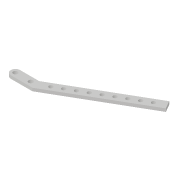
# Autodesk Inventor part: CollectorArmParametric
Saved by Autodesk Inventor 2018 (Build 220112000, 112)
## iProperties
Created: 2018-12-15
Part Number: CollectorArmParametric
Material: Generic
Document SubType Name: Modeling
Designer: ball
Density: 1 g/cm^3
Appearance: Default
Author: ball
Autodesk Inventor part; units mm, degrees
ref_plane "YZ Plane" through (0, 0, 0) normal (1, 0, 0) x (0, 1, 0)
ref_plane "XZ Plane" through (0, 0, 0) normal (0, 1, 0) x (-1, 0, 0)
ref_plane "XY Plane" through (0, 0, 0) normal (0, 0, 1) x (1, 0, 0)
sketch "Sketch1" plane through (0, 0, 0) normal (0, 1, 0) x (-1, 0, 0)
  line L0 (0, 0) -> (22.5298, 0)
  line L1 (22.5298, -9.525) -> (0, -9.525)
  line L2 (0, -9.525) -> (0, 0)
  arc A0 (22.5298, -9.525) -> (22.5298, 0) centre (22.5298, -4.7625) ccw
  line L3 (0, 0) -> (-87.9882, -50.8)
  line L4 (0, 0) -> (101.6, 0) construction
  line L5 (-87.9882, -50.8) -> (-83.2257, -59.0489)
  line L6 (0, 0) -> (4.7625, -8.2489)
  line L7 (4.7625, -8.2489) -> (-83.2257, -59.0489)
  circle A1 centre (22.5298, -4.7625) radius 2.2479
  line L8 (22.5298, -4.7625) -> (6.5278, -4.7625) construction
  circle A2 centre (6.5278, -4.7625) radius 2.2479
  line L9 (2.3813, -4.1244) -> (-8.6173, -10.4744) construction
  circle A3 centre (-8.6173, -10.4744) radius 1.9685
  line L10 (2.3813, -4.1244) -> (-85.6069, -54.9244) construction
  circle A4 centre (-17.0861, -15.3639) radius 1.9685
  circle A5 centre (-25.555, -20.2534) radius 1.9685
  circle A6 centre (-34.0239, -25.1429) radius 1.9685
  circle A7 centre (-42.4927, -30.0324) radius 1.9685
  circle A8 centre (-50.9616, -34.9219) radius 1.9685
  circle A9 centre (-59.4304, -39.8114) radius 1.9685
  circle A10 centre (-67.8993, -44.7009) radius 1.9685
  circle A11 centre (-76.3682, -49.5904) radius 1.9685
  line L11 (22.5298, -4.7625) -> (6.5278, -4.7625) construction
  line L12 (6.5278, -4.7625) -> (6.5278, 11.2395) construction
  line L13 (6.5278, 11.2395) -> (22.5298, 11.2395) construction
  line L14 (22.5298, 11.2395) -> (22.5298, -4.7625) construction
  line L15 (14.5288, 11.2395) -> (14.5288, -4.7625) construction
  line L16 (22.5298, 3.2385) -> (6.5278, 3.2385) construction
  circle A12 centre (14.5288, 3.2385) radius 1.27 construction
  dimension "d0" = 22.5298
  dimension "d1" = 9.525
  dimension "d2" = 4.7625
  dimension "d4" = 150
  dimension "d7" = 9.525
  dimension "d8" = 9.525
  dimension "d9" = 4.4958
  dimension "d10" = 16.002
  dimension "d11" = 4.4958
  dimension "d12" = 12.7
  dimension "d13" = 3.937
  dimension "d14" = 4.7625
  dimension "d15" = 3.937
  dimension "d16" = 9.779
  dimension "d17" = 3.937
  dimension "d18" = 9.779
  dimension "d19" = 3.937
  dimension "d20" = 9.779
  dimension "d21" = 3.937
  dimension "d22" = 9.779
  dimension "d23" = 3.937
  dimension "d24" = 9.779
  dimension "d25" = 3.937
  dimension "d26" = 9.779
  dimension "d27" = 3.937
  dimension "d28" = 9.779
  dimension "d29" = 3.937
  dimension "d30" = 9.779
  dimension "d31" = 16.002
  dimension "d32" = 2.54
  dimension "d33" = 115.8874
  constraints: 32 end point, 13 centre point, 7 midpoint, 4 horizontal, 3 coincident, 3 parallel, 3 perpendicular, 2 point on circle, 1 equal length, 11 other
  measures "d0" distance of L1.start L1.end
  measures "d1" distance of L0.end L1.start
  measures "d2" radius of A0
  measures "d4" angle of L3 L4
  measures "d7" distance of L5.end L3.end
  measures "d8" distance of L0.start L6.end
  measures "d9" diameter of A1
  measures "d10" distance of L8.start L8.end
  measures "d11" diameter of A2
  measures "d12" distance of L9.start L9.end
  measures "d13" diameter of A3
  measures "d14" distance from line of L3 L9.end
  measures "d15" diameter of A4
  measures "d16" distance of A4.centre L9.end
  measures "d17" diameter of A5
  measures "d18" distance of A5.centre A4.centre
  measures "d19" diameter of A6
  measures "d20" distance of A6.centre A5.centre
  measures "d21" diameter of A7
  measures "d22" distance of A7.centre A6.centre
  measures "d23" diameter of A8
  measures "d24" distance of A8.centre A7.centre
  measures "d25" diameter of A9
  measures "d26" distance of A9.centre A8.centre
  measures "d27" diameter of A10
  measures "d28" distance of A10.centre A9.centre
  measures "d29" diameter of A11
  measures "d30" distance of A11.centre A10.centre
  measures "d31" distance of L11.end L12.end
  measures "d32" diameter of A12
  measures "d33" distance of L3.end A12.centre
extrude "Extrusion1" add sketch "Sketch1" along normal blind 3.175
body "Solid1"
